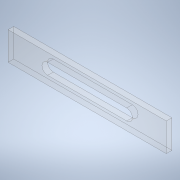
# Autodesk Inventor part: Electronics Side Plate
Saved by Autodesk Inventor 2022 (Build 260153000, 153)
## iProperties
Created: 2022-01-15
Part Number: Electronics Side Plate
Material: Generic
Document SubType Name: Modeling
Designer: merky
Density: 1 g/cm^3
Appearance: Polycarbonate - Clear
Author: merky
Autodesk Inventor part; units mm, degrees
ref_plane "YZ Plane" through (0, 0, 0) normal (1, 0, 0) x (0, 1, 0)
ref_plane "XZ Plane" through (0, 0, 0) normal (0, 1, 0) x (-1, 0, 0)
ref_plane "XY Plane" through (0, 0, 0) normal (0, 0, 1) x (1, 0, 0)
sketch "Sketch1" plane through (0, 0, 0) normal (0, 0, 1) x (1, 0, 0)
  line L0 (0, 0) -> (355.6, 0)
  line L1 (355.6, 0) -> (355.6, 63.5)
  line L2 (355.6, 63.5) -> (0, 63.5)
  line L3 (0, 63.5) -> (0, 0)
  line L4 (88.9, 31.75) -> (266.7, 31.75) construction
  line L5 (88.9, 19.05) -> (266.7, 19.05)
  line L6 (266.7, 44.45) -> (88.9, 44.45)
  arc A0 (88.9, 44.45) -> (88.9, 19.05) centre (88.9, 31.75) ccw
  arc A1 (266.7, 19.05) -> (266.7, 44.45) centre (266.7, 31.75) ccw
  point P0 (177.8, 31.75)
  dimension "d0" = 355.6
  dimension "d1" = 63.5
  dimension "d4" = 25.4
  dimension "d5" = 177.8
  dimension "d6" = 177.8
  constraints: 16 end point, 4 point on circle, 4 tangent, 3 parallel, 2 centre point, 2 horizontal, 1 midpoint, 1 perpendicular
  measures "d0" distance of L2.end L1.end
  measures "d1" distance of L1.end L0.end
  measures "d4" diameter of A1
  measures "d5" distance from line of L1 point (177.8, 31.75)
  measures "d6" distance of L6.start L6.end
extrude "Extrusion1" add sketch "Sketch1" along normal blind 12.7
body "Solid1"
